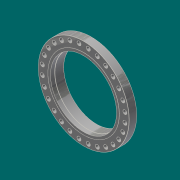
# Autodesk Inventor part: A1-19027-300-03 30in CL300 RF flange
Saved by Autodesk Inventor 2017.3 (Build 213256000, 256)
## iProperties
Created: 2011-05-31
Part Number: A1-19027-300-03 30in CL300 RF flange
Document SubType Name: Modeling
Designer: Graeme_Van_Dongen
Density: 7.85 g/cm^3
Description: 30" ASME B16.47 Ser.A CLASS 300 RFSO FLANGE, A105N
Material: Steel
Mass: 327253 g
Surface Area: 20036.2 cm^2
Volume: 41688.2 cm^3
Appearance: Steel
Author: Graeme_Van_Dongen
Autodesk Inventor part; units mm, degrees
ref_plane "YZ Plane" through (0, 0, 0) normal (1, 0, 0) x (0, 1, 0)
ref_plane "XZ Plane" through (0, 0, 0) normal (0, 1, 0) x (-1, 0, 0)
ref_plane "XY Plane" through (0, 0, 0) normal (0, 0, 1) x (1, 0, 0)
sketch "Sketch1" plane through (0, 0, 0) normal (0, 0, 1) x (1, 0, 0)
  circle A0 centre (0, 0) radius 546.1
  circle A1 centre (0, 0) radius 393.7
  dimension "d0" = 1092.2
  dimension "d1" = 787.4
  constraints: 2 centre point, 2 coincident
  measures "d0" diameter of A0
  measures "d1" diameter of A1
extrude "Extrusion1" add sketch "Sketch1" along normal blind 92.075
sketch "Sketch2" plane through (0, 0, 92.075) normal (0, 0, 1) x (1, 0, 0)
  circle A0 centre (0, 0) radius 393.7 projected
  circle A1 centre (0, 0) radius 546.1 projected
  circle A2 centre (0, 0) radius 428.625
  dimension "d4" = 857.25
  constraints: 1 centre point, 1 coincident
  measures "d4" diameter of A2
extrude "Extrusion2" add sketch "Sketch2" along normal blind 1.5875 contours A2
sketch "Sketch3" plane through (0, 0, 0) normal (0, 0, -1) x (-1, 0, 0)
  circle A0 centre (0, 0) radius 393.7 projected
  circle A1 centre (0, 0) radius 546.1 projected
  circle A2 centre (0, 0) radius 441.325
  dimension "d7" = 882.65
  constraints: 1 centre point, 1 coincident
  measures "d7" diameter of A2
extrude "Extrusion3" add sketch "Sketch3" along normal blind 61.9125 contours A2
sketch "Sketch4" plane through (0, 0, 93.6625) normal (0, 0, 1) x (1, 0, 0)
  circle A0 centre (0, 0) radius 428.625 projected
  line L0 (0, -764.54) -> (0, 764.54) projected
  line L1 (-764.54, 0) -> (764.54, 0) projected
  line L2 (0, 0) -> (55.8115, 495.3407) construction
  dimension "d13" = 498.475
  dimension "d14" = 6.429
  constraints: 2 end point
  measures "d13" distance of L2.start L2.end
  measures "d14" angle of L0 L2
hole "Hole1" at (55.8115, 495.3407, 93.6625) direction (0, 0, -1) diameter 47.625 end through all
chamfer "Chamfer3" distance 0.7937 angle 45 2 edges at (55.8115, 519.1532, 0) (55.8115, 519.1532, 92.075)
pattern_circular "Circular Pattern1" count 28 over 360 about axis through (0, 0, -10) along (0, 0, -1) of "Hole1", "Chamfer3"
chamfer "Chamfer2" distance 1.5875 angle 45 2 edges at (-546.1, 0, 92.075) (-546.1, 0, 0)
fillet "Fillet2" radius 11.1125 1 edges at (441.325, 0, 0)
chamfer "Chamfer4" distance 1.5875 angle 45 1 edges at (441.325, 0, -61.9125)
sketch "Sketch6" plane through (0, 0, 0) normal (1, 0, 0) x (0, 1, 0)
  line L0 (441.325, -11.1125) -> (441.325, -60.325) construction
  line L1 (439.7375, -61.9125) -> (-439.7375, -61.9125) construction
  line L2 (0, -93.0275) -> (0, 124.7775) projected
  line L3 (393.7, -61.9125) -> (393.7, 93.6625) construction
  line L4 (396.875, 93.6625) -> (396.875, 42.8625)
  line L5 (396.875, 42.8625) -> (393.7, 42.8625)
  line L6 (393.7, 42.8625) -> (393.7, 93.6625)
  line L7 (441.325, -33.3375) -> (441.325, -61.9125)
  line L8 (441.325, -61.9125) -> (395.2875, -61.9125)
  line L9 (395.2875, -61.9125) -> (406.4, -53.3856)
  line L10 (406.4, -53.3856) -> (406.4, -46.0375)
  arc A0 (419.1, -33.3375) -> (406.4, -46.0375) centre (419.1, -46.0375) ccw
  line L11 (419.1, -33.3375) -> (441.325, -33.3375)
  line L12 (393.7, 93.6625) -> (396.875, 93.6625)
  point P0 (0, 0)
  dimension "d71" = 50.8
  dimension "d72" = 396.875
  dimension "d94" = 406.4
  dimension "d95" = 11.1125
  dimension "d96" = 37.5
  dimension "d99" = 12.7
  dimension "d100" = 15.875
  dimension "d101" = 7.3481
  constraints: 19 end point, 4 point on line, 2 collinear, 2 perpendicular, 2 point on circle, 2 tangent, 1 centre point, 1 horizontal, 1 parallel, 1 vertical
  measures "d71" distance from line of L3.end L5
  measures "d72" distance from line of point (0, 0) L4
  measures "d94" distance between parallel lines of L2 L10
  measures "d95" horizontal distance of L8.end L9.end
  measures "d96" angle of L8 L9
  measures "d99" radius of A0
  measures "d100" distance from line of L8 A0.centre
  measures "d101" distance of L9.end L10.end
revolve "Revolution1" cut sketch "Sketch6" angle 360 about axis through (0, 0, -10) along (0, 0, 1)
fillet "Fillet5" radius 0.7937 1 edges at (0, -396.875, 42.8625)
equation "\"d0\" = OD"
equation "\"d1\" = Bore"
equation "\"d2\" = Thickness"
equation "\"d4\" = RFDia"
equation "\"d5\" = RFDepth"
equation "\"d7\" = NeckDia"
equation "\"d8\" = NeckLength"
equation "\"d13\" = 0.5 * BCD"
equation "\"d15\" = HoleDia"
equation "\"d30\" = HoleChamfer"
equation "\"d25\" = RimChamfer"
equation "\"d29\" = NeckFillet"
equation "\"d33\" = NeckChamfer"
equation "\"OD\" = 1092.2"
equation "\"Bore\" = 787.4"
equation "\"Thickness\" = 92.075"
equation "\"RFDia\" = 857.25"
equation "\"RFDepth\" = 1.5875"
equation "\"HoleDia\" = 47.625"
equation "\"BCD\" = 996.95"
equation "\"NeckDia\" = 882.65"
equation "\"NeckLength\" = 61.9125"
equation "\"HoleChamfer\" = 0.79375"
equation "\"RimChamfer\" = 1.5875"
equation "\"NeckChamfer\" = 1.5875"
equation "\"NeckFillet\" = 11.1125"
equation "\"Lock\" = 25.4"
equation "\"Lockstep\" = 3.175"
equation "\"Casing\" = 812.8"
equation "\"Size\" = 762"
equation "\"Wall\" = 12.7"
body "Solid1"
